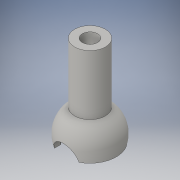
# Autodesk Inventor part: MatthewSheehan Caster
Saved by Autodesk Inventor 2016 (Build 200138000, 138)
## iProperties
Created: 2016-10-14
Part Number: MatthewSheehan Caster
Material: Generic
Document SubType Name: Modeling
Designer: MHSLibrary
Density: 1 g/cm^3
Appearance: Default
Author: MHSLibrary
Autodesk Inventor part; units mm, degrees
ref_plane "YZ Plane" through (0, 0, 0) normal (1, 0, 0) x (0, 1, 0)
ref_plane "XY Plane" through (0, 0, 0) normal (0, 0, 1) x (1, 0, 0)
sketch "Sketch1" plane through (0, 0, 0) normal (0, 1, 0) x (-1, 0, 0)
  circle A0 centre (0, 0) radius 6.35
  dimension "d0" = 12.7
  constraints: 1 centre point, 1 coincident
  measures "d0" diameter of A0
extrude "Extrusion2" add sketch "Sketch1" along normal blind 76.2
ref_plane "Work Plane1" through (0, -3.175, 0) normal (0, 1, 0) x (-1, 0, 0)
sketch "Sketch9" plane through (0, 76.2, 0) normal (0, 1, 0) x (1, 0, 0)
  circle A0 centre (0, 0) radius 3.175
  dimension "d22" = 6.35
  constraints: 1 centre point, 1 coincident
  measures "d22" diameter of A0
ref_plane "Work Plane2" through (0, 71.501, 0) normal (0, 1, 0) x (1, 0, 0)
sketch "Sketch10" plane through (0, 71.501, 0) normal (0, 1, 0) x (1, 0, 0)
  circle A0 centre (0, 0) radius 2.921
  dimension "d24" = 5.842
  constraints: 1 centre point, 1 coincident
  measures "d24" diameter of A0
loft "Loft1" cut profiles "Sketch9", "Sketch10"
sketch "Sketch11" plane through (0, 0, 0) normal (0, -1, 0) x (1, 0, 0)
  circle A0 centre (0, 0) radius 9.144
  line L0 (0, 9.144) -> (0, -9.144)
  dimension "d29" = 18.288
  constraints: 2 end point, 2 point on circle, 1 centre point, 1 coincident, 1 vertical
  measures "d29" diameter of A0
sketch "Sketch15" plane through (0, 0, 0) normal (0, -1, 0) x (1, 0, 0)
  circle A0 centre (0, 0) radius 11.2891
  line L0 (11.2891, 0) -> (-11.2891, 0)
  constraints: 2 end point, 2 point on circle, 1 centre point, 1 coincident, 1 horizontal
revolve "Revolution8" add sketch "Sketch15" angle 360 about axis through (11.2891, 0, 0) along (-1, 0, 0)
revolve "Revolution9" cut sketch "Sketch11" angle 360 about axis through (0, 0, 9.144) along (0, 0, -1)
ref_plane "Work Plane4" through (0, -3.1115, 0) normal (0, 1, 0) x (1, 0, 0)
sketch "Sketch16" plane through (0, -3.1115, 0) normal (0, 1, 0) x (1, 0, 0)
  circle A0 centre (0, 0) radius 28.2257
  line L0 (28.2257, 0) -> (-28.2257, 0)
  constraints: 2 end point, 2 point on circle, 1 centre point, 1 coincident, 1 horizontal
revolve "Revolution10" cut sketch "Sketch16" angle 180 about axis through (28.2257, -3.1115, 0) along (1, 0, 0) picked at (-5.3447, -7.7431) contours A0 L0
sketch "Sketch17" plane through (0, 0, 0) normal (0, 0, 1) x (1, 0, 0)
  line L0 (-8.5983, -3.1115) -> (8.5983, -3.1115) projected
  circle A0 centre (0, -3.1115) radius 5.0587
  point P0 (0, 0)
  constraints: 1 centre point, 1 midpoint
extrude "Extrusion7" cut sketch "Sketch17" along normal mid plane 25.4
ref_plane "Work Plane8" through (0, 34.0233, 0) normal (0, 1, 0) x (-1, 0, 0)
ref_plane "Work Plane7" through (0, -3.1115, 0) normal (0, 1, 0) x (-1, 0, 0)
sketch "Sketch18" plane through (0, 34.0233, 0) normal (0, 1, 0) x (-1, 0, 0)
  circle A0 centre (0, 0) radius 6.35
  constraints: 1 centre point, 1 coincident
extrude "Extrusion8" cut sketch "Sketch18" along normal blind 50.8
sketch "Sketch19" plane through (0, 34.0233, 0) normal (0, 1, 0) x (1, 0, 0)
  circle A0 centre (0, 0) radius 6.35 projected
  circle A1 centre (0, 0) radius 3.175
  dimension "d51" = 6.35
  constraints: 1 centre point, 1 coincident
  measures "d51" diameter of A1
ref_plane "Work Plane9" through (0, 29.3243, 0) normal (0, 1, 0) x (-1, 0, 0)
sketch "Sketch20" plane through (0, 29.3243, 0) normal (0, 1, 0) x (-1, 0, 0)
  circle A0 centre (0, 0) radius 2.921
  dimension "d53" = 5.842
  constraints: 1 centre point, 1 coincident
  measures "d53" diameter of A0
loft "Loft2" cut profiles "Sketch20", "Sketch19" contours all / A1
body "Solid2"
